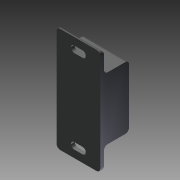
# Autodesk Inventor part: MGCE15-5
Saved by Autodesk Inventor 2011 SP1 (Build 150282100, 282)
## iProperties
Created: 2015-02-01
Part Number: MGCE15-5
Catalog Web Link: www.cadenas.de
Description: MGCE1-MAgnet Catches for Frames - Magnet
Vendor: MISUMI
Document SubType Name: Modeling
Designer: PARTuser1
Manufacturer: MISUMI
Mass: 13.3957 g
Surface Area: 46.414 cm^2
Volume: 13.3957 cm^3
Density: 1 g/cm^3
Category: PARTsolutions
Company: MISUMI
Title: MGCE15-5
Author: Cadenas PARTsolutions
Comments: MAgnet Catches for Frames - Magnet
PSOL_IDENT_0: {\\10.0.0.236\data_v8\23d-libs\misumi\metric\39_accessories_for_al_extrusions\hmgce_magnet.prj},157
PSOL_IDENT_1: {VTYP=3D},{NB=MGCE15-5},{LINA=MGCE15-5},{NN=MGCE1},{DATE=17.11.2014 05:31:13},{GEOMDATE=17.12.2009 0
PSOL_IDENT_2: 0:00:00},{VERSION=},{LINEID=10},{LINESUBID=-1},{WBVAR=}  {NB=MGCE15-5},{LINA=MGCE15-5},{KT=DUMMY},{P
PSOL_IDENT_3: N=MGCE15-5},{TYPE=MGCE1},{MATH=Aluminum Alloy},{STH=Alumite Treatment},{MATM=Feritte},{MATAB=Low Car
PSOL_IDENT_4: bon Steel},{STAB=Nickel Plating},{NO=5-5},{MG=MGCE1},{PL=ME5-5},{FRBOLT=SCB4-6},{FRBOLTQ=2},{FRNUT=H
PSOL_IDENT_5: NTT5-4},{FRNUTQ=2},{FRSCREW=SCB3-6},{FRSCREWQ=2},{DSCREW=HFBCM3-6},{DSCREWQ=2},{NUT=HNTT5-3}
SUPPLIER: MISUMI
ARTICLENO: MGCE15-5
BOMINFO: MGCE15-5
CREATOR: CADENAS GmbH
Autodesk Inventor part; units mm, degrees
sketch "Sketch_2" plane through (0, 0, 0) normal (0, 1, 0) x (-1, 0, 0)
  line L0 (0, -26.25) -> (0, 26.25)
  arc A0 (0, 26.25) -> (-2, 28.25) centre (-2, 26.25) ccw
  line L1 (-2, 28.25) -> (-21.5, 28.25)
  arc A1 (-21.5, 28.25) -> (-23.5, 26.25) centre (-21.5, 26.25) ccw
  line L2 (-23.5, 26.25) -> (-23.5, -26.25)
  arc A2 (-23.5, -26.25) -> (-21.5, -28.25) centre (-21.5, -26.25) ccw
  line L3 (-21.5, -28.25) -> (-2, -28.25)
  arc A3 (-2, -28.25) -> (0, -26.25) centre (-2, -26.25) ccw
  arc A4 (-9.5, 20.75) -> (-9.5, 24.25) centre (-9.5, 22.5) ccw
  line L4 (-9.5, 24.25) -> (-14, 24.25)
  arc A5 (-14, 24.25) -> (-14, 20.75) centre (-14, 22.5) ccw
  line L5 (-14, 20.75) -> (-9.5, 20.75)
  arc A6 (-9.5, -24.25) -> (-9.5, -20.75) centre (-9.5, -22.5) ccw
  line L6 (-9.5, -20.75) -> (-14, -20.75)
  arc A7 (-14, -20.75) -> (-14, -24.25) centre (-14, -22.5) ccw
  line L7 (-14, -24.25) -> (-9.5, -24.25)
  constraints: 16 end point, 16 point on circle, 8 centre point
extrude "Extrusion1" add sketch "Sketch_2" along normal blind 15.5
sketch "Sketch_1" plane through (0, 0, 0) normal (1, 0, 0) x (0, 1, 0)
  line L0 (-10, 50) -> (-10, -50)
  line L1 (-10, -50) -> (30, -50)
  line L2 (30, -50) -> (30, 50)
  line L3 (30, 50) -> (-10, 50)
  line L4 (0, 28.25) -> (0, -28.25)
  arc A0 (0, -28.25) -> (2, -26.25) centre (0, -26.25) ccw
  line L5 (2, -26.25) -> (2, -18.75)
  arc A1 (4, -16.75) -> (2, -18.75) centre (4, -18.75) ccw
  line L6 (4, -16.75) -> (13.5, -16.75)
  arc A2 (13.5, -16.75) -> (15.5, -14.75) centre (13.5, -14.75) ccw
  line L7 (15.5, -14.75) -> (15.5, 14.75)
  arc A3 (15.5, 14.75) -> (13.5, 16.75) centre (13.5, 14.75) ccw
  line L8 (13.5, 16.75) -> (4, 16.75)
  arc A4 (2, 18.75) -> (4, 16.75) centre (4, 18.75) ccw
  line L9 (2, 18.75) -> (2, 26.25)
  arc A5 (2, 26.25) -> (0, 28.25) centre (0, 26.25) ccw
  constraints: 20 end point, 12 point on circle, 6 centre point
extrude "Extrusion2" cut sketch "Sketch_1" along normal blind 24
sketch "Sketch_3" plane through (0, 0, 0) normal (1, 0, 0) x (0, 1, 0)
  line L0 (3, 10.75) -> (3, -10.75)
  line L1 (3, -10.75) -> (5, -10.75)
  line L2 (5, -10.75) -> (5, 10.75)
  line L3 (5, 10.75) -> (3, 10.75)
  constraints: 8 end point
extrude "Extrusion3" add sketch "Sketch_3" against normal blind 3
sketch "Sketch_4" plane through (0, 0, 0) normal (1, 0, 0) x (0, 1, 0)
  line L0 (11.5, 10.75) -> (11.5, -10.75)
  line L1 (11.5, -10.75) -> (13.5, -10.75)
  line L2 (13.5, -10.75) -> (13.5, 10.75)
  line L3 (13.5, 10.75) -> (11.5, 10.75)
  constraints: 8 end point
extrude "Extrusion4" add sketch "Sketch_4" against normal blind 3
ref_plane "magnet_to_mgplate_XY" through (-3, 8, 0) normal (1, 0, 0) x (0, 0, -1)
ref_plane "magnet_to_mgplate_YZ" through (-3, 8, 0) normal (0, 0, -1) x (0, 1, 0)
ref_plane "magnet_to_mgplate_ZX" through (-3, 8, 0) normal (0, 1, 0) x (1, 0, 0)
ref_plane "to_plate_XY" through (11.9, 0, -22.5) normal (0, 1, 0) x (1, 0, 0)
ref_plane "to_plate_YZ" through (11.9, 0, -22.5) normal (1, 0, 0) x (0, 0, -1)
ref_plane "to_plate_ZX" through (11.9, 0, -22.5) normal (0, 0, -1) x (0, 1, 0)
body "Solid1"
